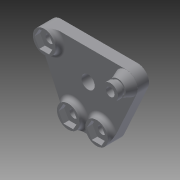
# Autodesk Inventor part: lamp_trap_2
Saved by Autodesk Inventor 2013 (Build 170138000, 138)
## iProperties
Created: 2013-02-11
Part Number: lamp_trap_2
Material: Generic
Document SubType Name: Modeling
Designer: Brad
Density: 1 g/cm^3
Author: Brad
Autodesk Inventor part; units mm, degrees
ref_plane "YZ Plane" through (0, 0, 0) normal (1, 0, 0) x (0, 1, 0)
ref_plane "XZ Plane" through (0, 0, 0) normal (0, 1, 0) x (-1, 0, 0)
ref_plane "XY Plane" through (0, 0, 0) normal (0, 0, 1) x (1, 0, 0)
sketch "Sketch1" plane through (0, 0, 0) normal (0, 0, 1) x (1, 0, 0)
  circle A0 centre (0, 0) radius 3.5
  line L0 (0, 0) -> (7.5, 0)
  line L1 (0, 0) -> (-7.5, 0)
  line L2 (7.5, 0) -> (7.5, -18.108285)
  line L3 (-7.5, 0) -> (-7.5, -18.108285)
  circle A1 centre (7.5, -18.108285) radius 2.25
  circle A2 centre (-7.5, -18.108285) radius 2.25
  circle A3 centre (0, 0) radius 22.5
  line L4 (0, 0) -> (20.25, 0)
  line L5 (20.25, 0) -> (20.25, 9.807523)
  line L6 (0, 0) -> (-20.25, 0)
  line L7 (-20.25, 0) -> (-20.25, 9.807523)
  circle A4 centre (20.25, 9.807523) radius 2.25
  circle A5 centre (-20.25, 9.807523) radius 2.25
  line L8 (-20.25, 9.807523) -> (20.25, 9.807523)
  line L9 (20.25, 9.807523) -> (7.5, -18.108285)
  line L10 (7.5, -18.108285) -> (-7.5, -18.108285)
  line L11 (-7.5, -18.108285) -> (-20.25, 9.807523)
  line L12 (-20.25, 15.807523) -> (20.25, 15.807523)
  line L13 (25.707698, 7.314826) -> (12.957698, -20.600982)
  line L14 (7.5, -24.108285) -> (-7.5, -24.108285)
  line L15 (-12.957698, -20.600982) -> (-25.707698, 7.314826)
  circle A6 centre (-20.25, 9.807523) radius 6
  circle A7 centre (20.25, 9.807523) radius 6
  circle A8 centre (7.5, -18.108285) radius 6
  arc A9 (-13.499036, -18.000723) -> (-7.5, -24.108285) centre (-7.5, -18.108285) ccw
  arc A10 (-7.5, -18.108285) -> (7.5, -18.108285) centre (0, 0) ccw
  dimension "d0" = 7
  dimension "d1" = 7.5
  dimension "d2" = 7.5
  dimension "d4" = 4.5
  dimension "d5" = 4.5
  dimension "d6" = 45
  dimension "d7" = 20.25
  dimension "d8" = 20.25
  dimension "d9" = 4.5
  dimension "d10" = 4.5
  dimension "d11" = 6
  dimension "d27" = 12
  dimension "d28" = 6
  dimension "d29" = 12
  dimension "d30" = 12
  constraints: 32 end point, 14 point on circle, 11 centre point, 9 coincident, 4 perpendicular, 4 tangent, 2 equal length, 1 horizontal, 1 point on line
  measures "d0" diameter of A0
  measures "d1" distance of L0.start L0.end
  measures "d2" distance of L0.start L1.end
  measures "d4" diameter of A1
  measures "d5" diameter of A2
  measures "d6" diameter of A3
  measures "d7" distance of L4.start L4.end
  measures "d8" distance of L4.start L6.end
  measures "d9" diameter of A4
  measures "d10" diameter of A5
  measures "d11" distance between parallel lines of L8 L12
  measures "d27" diameter of A8
  measures "d28" radius of A9
  measures "d29" diameter of A6
  measures "d30" diameter of A7
extrude "Extrusion1" add sketch "Sketch1" along normal blind 6 contours L0 L2 A8 L10 A2 L3 L1 A0 | A0 L1 L6 L11 A6 L8 A7 L9 L4 L0 | L4 L9 A8 L2 | L3 A2 L11 L6 | A8 L9 A1 L2 | L2 A1 L10 A8 | L9 A7 L5 L4 | L4 L5 A7 A3 L13 A8 L9 | L11 A2 A10 A8 A3 L15 A6 L7 L6 | L6 L7 A6 L11 | A8 A3 A10 A1 L9 | A8 A10 A2 L10 | L10 A1 A10 A8 | A7 L8 A4 L9 | L9 A4 L5 A7 | A6 L7 A5 L11 | L11 A5 L8 A6 | A8 A3 | A3 L13 A8 | L5 A4 A3 A7 | A7 A3 A4 L8 | L8 A6 A3 L12 A7 | A6 A3 A5 L7 | L8 A5 A3 A6 | A8 L14 A9 A3 | A7 L13 A3 | A3 A4 A7 | A3 L12 A7 | A6 A3 A5 | A3 L15 A6 | A6 L12 A3 | A9 L15 A3
sketch "Sketch2" plane through (0, 0, 0) normal (0, 0, -1) x (-1, 0, 0)
  circle A0 centre (0, 0) radius 3.5 projected
  circle A1 centre (0, 0) radius 6.5
  circle A2 centre (0, 0) radius 3.5
  dimension "d14" = 13
  constraints: 2 centre point, 2 coincident, 1 concentric
  measures "d14" diameter of A1
extrude "Extrusion2" add sketch "Sketch2" along normal blind 4.5
fillet "Fillet1" radius 3 1 edges at (6.5, 0, 0)
sketch "Sketch7" plane through (0, 0, 6) normal (0, 0, 1) x (1, 0, 0)
  circle A0 centre (20.25, 9.807523) radius 2.25
  arc A1 (25.707698, 7.314826) -> (20.25, 15.807523) centre (20.25, 9.807523) ccw
  circle A2 centre (20.25, 9.807523) radius 4.125
  dimension "d38" = 8.25
  constraints: 1 centre point, 1 coincident
  measures "d38" diameter of A2
extrude "Extrusion7" add sketch "Sketch7" along normal blind 4.5
sketch "Sketch8" plane through (20.25, 9.807523, 10.5) normal (0, 0, 1) x (1, 0, 0)
  circle A0 centre (0, 0) radius 2.25 projected
  circle A1 centre (0, 0) radius 4.125 projected
  circle A2 centre (0, 0) radius 3.5
  point P0 (-20.25, -9.807523)
  dimension "d41" = 7
  constraints: 1 centre point, 1 coincident
  measures "d41" diameter of A2
extrude "Extrusion8" add sketch "Sketch8" along normal blind 1.5 contours A2
sketch "Sketch9" plane through (20.25, 9.807523, 12) normal (0, 0, 1) x (1, 0, 0)
  circle A0 centre (0, 0) radius 2.25 projected
  circle A1 centre (0, 0) radius 3.5 projected
  circle A2 centre (0, 0) radius 4.125
  point P0 (-20.25, -9.807523)
  dimension "d44" = 8.25
  constraints: 1 centre point, 1 coincident
  measures "d44" diameter of A2
extrude "Extrusion9" add sketch "Sketch9" along normal blind 2.5 contours A1 | A2
draft "FaceDraft2" angle 22 pull direction (0, 0, 1) faces at (24.361624, 9.475598, 9) fixed edges at (16.125, 9.807523, 10.5)
sketch "Sketch10" plane through (0, 0, 6) normal (0, 0, 1) x (1, 0, 0)
  arc A0 (-20.25, 15.807523) -> (-25.707698, 7.314826) centre (-20.25, 9.807523) ccw
  line L0 (-15.053848, 9.807523) -> (-17.651924, 5.307523)
  line L1 (-17.651924, 5.307523) -> (-22.848076, 5.307523)
  line L2 (-22.848076, 5.307523) -> (-25.446152, 9.807523)
  line L3 (-25.446152, 9.807523) -> (-22.848076, 14.307523)
  line L4 (-22.848076, 14.307523) -> (-17.651924, 14.307523)
  line L5 (-17.651924, 14.307523) -> (-15.053848, 9.807523)
  circle A1 centre (-20.25, 9.807523) radius 6
  line L6 (-2.303848, -18.108285) -> (-4.901924, -22.608285)
  line L7 (-4.901924, -22.608285) -> (-10.098076, -22.608285)
  line L8 (-10.098076, -22.608285) -> (-12.696152, -18.108285)
  line L9 (-12.696152, -18.108285) -> (-10.098076, -13.608285)
  line L10 (-10.098076, -13.608285) -> (-4.901924, -13.608285)
  line L11 (-4.901924, -13.608285) -> (-2.303848, -18.108285)
  circle A2 centre (-7.5, -18.108285) radius 6
  line L12 (12.696152, -18.108285) -> (10.098076, -22.608285)
  line L13 (10.098076, -22.608285) -> (4.901924, -22.608285)
  line L14 (4.901924, -22.608285) -> (2.303848, -18.108285)
  line L15 (2.303848, -18.108285) -> (4.901924, -13.608285)
  line L16 (4.901924, -13.608285) -> (10.098076, -13.608285)
  line L17 (10.098076, -13.608285) -> (12.696152, -18.108285)
  circle A3 centre (7.5, -18.108285) radius 6
  dimension "d48" = 9
  dimension "d49" = 9
  dimension "d50" = 9
  constraints: 36 end point, 3 centre point, 2 coincident, 1 concentric, 13 other
  measures "d48" distance between parallel lines of L1 L4
  measures "d49" distance between parallel lines of L7 L10
  measures "d50" distance between parallel lines of L13 L16
extrude "Extrusion10" add sketch "Sketch10" along normal blind 3
fillet "Fillet3" radius 2 6 edges at (-16.0074, 14.0502, 6) (-18.9745, 3.9447, 6) (-3.2574, -22.3509, 6) (-8.7755, -12.2454, 6) (13.3629, -19.3838, 6) (3.2574, -13.8656, 6)
body "Solid1"
